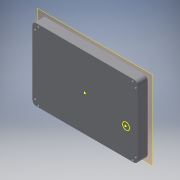
# Autodesk Inventor part: 03_Omniscope_lid_lenses
Saved by Autodesk Inventor 2019.4 (Build 234330000, 330)
## iProperties
Created: 2021-09-27
Part Number: 03_Omniscope_lid_lenses
Material: Generic
Document SubType Name: Modeling
Designer: diederichbenedict
Density: 1 g/cm^3
Appearance: Default
Author: diederichbenedict
Autodesk Inventor part; units mm, degrees
ref_plane "YZ Plane" through (0, 0, 0) normal (1, 0, 0) x (0, 1, 0)
ref_plane "XZ Plane" through (0, 0, 0) normal (0, 1, 0) x (-1, 0, 0)
ref_plane "XY Plane" through (0, 0, 0) normal (0, 0, 1) x (1, 0, 0)
ref_plane "Work Plane1" through (0, 0, 0) normal (0, 0, 1) x (1, 0, 0)
sketch "Sketch1" plane through (0, 0, 0) normal (0, 0, 1) x (1, 0, 0)
  circle A0 centre (-56, 33.5) radius 1.35 projected
  circle A1 centre (-52.5, -38) radius 1.35 projected
  circle A2 centre (56, -33.5) radius 1.35 projected
  circle A3 centre (52.5, 38) radius 1.35 projected
  circle A4 centre (56, 33.5) radius 1.35 projected
  circle A5 centre (52.5, -38) radius 1.35 projected
  circle A6 centre (-56, -33.5) radius 1.35 projected
  circle A7 centre (-52.5, 38) radius 1.35 projected
  line L0 (-54.4, 35.9) -> (54.4, 35.9) projected
  line L1 (54.4, 35.9) -> (54.4, -35.9) projected
  line L2 (54.4, -35.9) -> (-54.4, -35.9) projected
  line L3 (-54.4, -35.9) -> (-54.4, 35.9) projected
  arc A8 (-58.5, -36) -> (-54.5, -40) centre (-54.5, -36) ccw projected
  line L4 (-54.5, -40) -> (54.5, -40) projected
  arc A9 (54.5, -40) -> (58.5, -36) centre (54.5, -36) ccw projected
  line L5 (58.5, -36) -> (58.5, 36) projected
  arc A10 (58.5, 36) -> (54.5, 40) centre (54.5, 36) ccw projected
  line L6 (54.5, 40) -> (-54.5, 40) projected
  arc A11 (-54.5, 40) -> (-58.5, 36) centre (-54.5, 36) ccw projected
  line L7 (-58.5, 36) -> (-58.5, -36) projected
  point P0 (0, 0)
ref_plane "Work Plane2" through (41.5917, 22.95, 7) normal (0, 0, -1) x (0, 1, 0)
extrude "Extrusion1" add sketch "Sketch1" along normal up to surface (7 mm away)
sketch "Sketch2" plane through (-54.5, -40, 7) normal (0, 0, 1) x (1, 0, 0)
  line L0 (108.9, 75.9) -> (108.9, 4.1) projected
  line L1 (108.9, 4.1) -> (0.1, 4.1) projected
  line L2 (0.1, 4.1) -> (0.1, 75.9) projected
  line L3 (0.1, 75.9) -> (108.9, 75.9) projected
  circle A0 centre (2, 78) radius 1.35 projected
  circle A1 centre (-1.5, 6.5) radius 1.35 projected
  circle A2 centre (107, 2) radius 1.35 projected
  circle A3 centre (110.5, 73.5) radius 1.35 projected
  circle A4 centre (107, 78) radius 1.35 projected
  circle A5 centre (110.5, 6.5) radius 1.35 projected
  circle A6 centre (2, 2) radius 1.35 projected
  circle A7 centre (-1.5, 73.5) radius 1.35 projected
  line L4 (-4, 76) -> (-4, 4) projected
  arc A8 (-4, 4) -> (0, 0) centre (0, 4) ccw projected
  line L5 (0, 0) -> (109, 0) projected
  arc A9 (109, 0) -> (113, 4) centre (109, 4) ccw projected
  line L6 (113, 4) -> (113, 76) projected
  arc A10 (113, 76) -> (109, 80) centre (109, 76) ccw projected
  line L7 (109, 80) -> (0, 80) projected
  arc A11 (0, 80) -> (-4, 76) centre (0, 76) ccw projected
  point P0 (54.5, 40)
extrude "Extrusion2" add sketch "Sketch2" along normal blind 4 contours L0 L1 L2 L3 | A11 L7 A10 L6 A9 L5 A8 L4
sketch "Sketch3" plane through (-54.5, -40, 11) normal (0, 0, 1) x (1, 0, 0)
  circle A0 centre (99.9917, 30.85) radius 3.9 projected
  circle A1 centre (99.9917, 66.85) radius 4.2 projected
  circle A2 centre (99.9917, 66.85) radius 3.375
  point P0 (54.5, 40)
  dimension "d4" = 6.75
  constraints: 1 centre point, 1 coincident
  measures "d4" diameter of A2
extrude "Extrusion3" cut sketch "Sketch3" against normal through all contours A2
sketch "Sketch4" plane through (-54.5, -40, 7) normal (0, 0, -1) x (-1, 0, 0)
  circle A0 centre (-99.9917, 66.85) radius 1.4124 projected
  circle A1 centre (-99.9917, 66.85) radius 3.9 projected
  point P0 (-54.5, 40)
extrude "Extrusion4" cut sketch "Sketch4" against normal blind 1 contours A0 | A1
pattern_linear "Rectangular Pattern1" count 6 spacing 18 along (-1, 0, 0) count 4 spacing 18 along (0, -1, 0) of "Extrusion3", "Extrusion4"
sketch "Sketch5" plane through (-54.5, -40, 11) normal (0, 0, 1) x (1, 0, 0)
  circle A0 centre (9.9917, 12.85) radius 3.375 projected
  circle A1 centre (27.9917, 12.85) radius 3.375 projected
  circle A2 centre (45.9917, 12.85) radius 3.375 projected
  circle A3 centre (63.9917, 12.85) radius 3.375 projected
  circle A4 centre (81.9917, 12.85) radius 3.375 projected
  circle A5 centre (99.9917, 12.85) radius 3.375 projected
  circle A6 centre (9.9917, 30.85) radius 3.375 projected
  circle A7 centre (27.9917, 30.85) radius 3.375 projected
  circle A8 centre (45.9917, 30.85) radius 3.375 projected
  circle A9 centre (63.9917, 30.85) radius 3.375 projected
  circle A10 centre (81.9917, 30.85) radius 3.375 projected
  circle A11 centre (99.9917, 30.85) radius 3.375 projected
  circle A12 centre (9.9917, 48.85) radius 3.375 projected
  circle A13 centre (27.9917, 48.85) radius 3.375 projected
  circle A14 centre (45.9917, 48.85) radius 3.375 projected
  circle A15 centre (63.9917, 48.85) radius 3.375 projected
  circle A16 centre (81.9917, 48.85) radius 3.375 projected
  circle A17 centre (99.9917, 48.85) radius 3.375 projected
  circle A18 centre (9.9917, 66.85) radius 3.375 projected
  circle A19 centre (27.9917, 66.85) radius 3.375 projected
  circle A20 centre (45.9917, 66.85) radius 3.375 projected
  circle A21 centre (63.9917, 66.85) radius 3.375 projected
  circle A22 centre (81.9917, 66.85) radius 3.375 projected
  circle A23 centre (99.9917, 66.85) radius 3.375 projected
  circle A24 centre (-1.5, 73.5) radius 1.35 projected
  circle A25 centre (2, 2) radius 1.35 projected
  circle A26 centre (110.5, 6.5) radius 1.35 projected
  circle A27 centre (107, 78) radius 1.35 projected
  circle A28 centre (110.5, 73.5) radius 1.35 projected
  circle A29 centre (107, 2) radius 1.35 projected
  circle A30 centre (-1.5, 6.5) radius 1.35 projected
  circle A31 centre (2, 78) radius 1.35 projected
  line L0 (-4, 76) -> (-4, 4) projected
  arc A32 (-4, 4) -> (0, 0) centre (0, 4) ccw projected
  line L1 (0, 0) -> (109, 0) projected
  arc A33 (109, 0) -> (113, 4) centre (109, 4) ccw projected
  line L2 (113, 4) -> (113, 76) projected
  arc A34 (113, 76) -> (109, 80) centre (109, 76) ccw projected
  line L3 (109, 80) -> (0, 80) projected
  arc A35 (0, 80) -> (-4, 76) centre (0, 76) ccw projected
  point P0 (54.5, 40)
hole "Hole1" at (52.5, -38, 11) at (56, -33.5, 11) at (56, 33.5, 11) at (52.5, 38, 11) at (-52.5, -38, 11) at (-56, -33.5, 11) at (-56, 33.5, 11) at (-52.5, 38, 11) direction (0, 0, -1) diameter 2.8 depth 12 tip angle 118 counterbore diameter 6 counterbore depth 3
body "Solid1"
